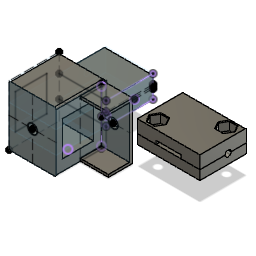
cessna-throttle-v39 (Autodesk Fusion 360 design; units mm, degrees)
Autodesk Fusion 360 part; units mm, degrees
note: some values were not read from the file. Chosen so that the rebuilt part matches the saved one: which bodies a step acts on.
sketch "Sketch1" plane through (0, 0, 0) normal (0, 1, 0) x (1, 0, 0)
  line L0 (0, 0) -> (20, 0)
  line L1 (20, 0) -> (20, 15)
  line L2 (20, 15) -> (0, 15)
  line L3 (0, 15) -> (0, 0)
  line L4 (6, 0) -> (6, 7)
  line L5 (6, 7) -> (14, 7)
  line L6 (14, 7) -> (14, 0)
  line L7 (10, 15) -> (10, 0) construction
  line L8 (0, 10) -> (20, 10) construction
  line L9 (20, 10) -> (20, 8.05) construction
  line L10 (20, 8.05) -> (0, 8.05) construction
  line L11 (0, 8.05) -> (0, 10) construction
  circle A0 centre (3.5, 3.05) radius 1
  circle A1 centre (16.5, 12) radius 1
  dimension "d1" = 7
  dimension "d2" = 8
  dimension "d3" = 20
  dimension "d4" = 15
  dimension "d5" = 1.95
  dimension "d6" = 5
  dimension "d7" = 2
  dimension "d8" = 3.5
  dimension "d9" = 5
  dimension "d10" = 2
  dimension "d11" = 2
  dimension "d12" = 3.5
  constraint horizontal L0
  constraint vertical L1
  constraint horizontal L2
  constraint vertical L3
  constraint coincident L0 L4.start
  constraint perpendicular L0 L4
  constraint perpendicular L4 L5
  constraint coincident L0 L6.end
  constraint perpendicular L0 L6
  constraint midpoint L2 L7.start
  constraint midpoint L0 L7.end
  constraint symmetric L4.end L5.end L7
  constraint coincident L0.start L3.end
  constraint horizontal L8
  constraint vertical L9
  constraint horizontal L10
  constraint vertical L11
  constraint coincident L1 L9.end
  constraint coincident L3 L8.start
  measures "d1" distance of L4.start L4.end
  measures "d2" distance of L4.end L5.end
  measures "d3" distance of L1.end L2.end
  measures "d4" distance of L0.start L2.end
  measures "d5" distance of L8 L10
  measures "d6" distance of L2 L8
  measures "d7" diameter of A0
  measures "d8" distance of L3 A0.centre
  measures "d9" distance of L10 A0.centre
  measures "d10" diameter of A1
  measures "d11" distance of L8 A1.centre
  measures "d12" distance of L1 A1.centre
extrude "Extrude1" add sketch "Sketch1" along normal blind 1.12 contours L0 L1 L2 L3 L4 L5 L6 makes body 1
sketch "Sketch2" plane through (0, 1.12, 0) normal (0, 1, 0) x (-1, 0, 0)
  circle A0 centre (-16.5, -12) radius 1
  circle A1 centre (-3.5, -3.05) radius 1
  line L0 (-14, -7) -> (-14, 0)
  line L1 (-14, 0) -> (-20, 0)
  line L2 (-20, 0) -> (-20, -15)
  line L3 (-20, -15) -> (0, -15)
  line L4 (0, -15) -> (0, 0)
  line L5 (0, 0) -> (-6, 0)
  line L6 (-6, 0) -> (-6, -7)
  line L7 (-6, -7) -> (-14, -7)
  line L8 (0, -15) -> (-20, -15)
  line L9 (-20, -15) -> (-20, 0)
  line L10 (-20, 0) -> (0, 0)
  line L11 (0, 0) -> (0, -15)
  constraint horizontal L8
  constraint vertical L9
  constraint horizontal L10
  constraint vertical L11
  constraint coincident L1.end L2.start
  constraint coincident L3.end L4.start
extrude "Extrude2" add sketch "Sketch2" along normal blind 3 bodies 1
sketch "Sketch3" plane through (0, 0, 0) normal (0, -1, 0) x (1, 0, 0)
  circle A0 centre (16.5, -12) radius 1
  circle A1 centre (3.5, -3.05) radius 1
  line L0 (14, 0) -> (14, -7)
  line L1 (14, -7) -> (6, -7)
  line L2 (6, -7) -> (6, 0)
  line L3 (6, 0) -> (0, 0)
  line L4 (0, 0) -> (0, -15)
  line L5 (0, -15) -> (20, -15)
  line L6 (20, -15) -> (20, 0)
  line L7 (20, 0) -> (14, 0)
  line L8 (0, 0) -> (20, 0)
  line L9 (20, 0) -> (20, -15)
  line L10 (20, -15) -> (0, -15)
  line L11 (0, -15) -> (0, 0)
  constraint horizontal L8
  constraint vertical L9
  constraint horizontal L10
  constraint vertical L11
  constraint coincident L5.end L6.start
  constraint coincident L3.end L4.start
extrude "Extrude3" add sketch "Sketch3" along normal blind 3 bodies 1
sketch "Sketch4" plane through (0, 0, 0) normal (-1, 0, 0) x (0, 0, 1)
  line L0 (0, -3) -> (0, 4.12)
  line L1 (0, 4.12) -> (-15, 4.12)
  line L2 (-15, 4.12) -> (-15, -3)
  line L3 (-15, -3) -> (0, -3)
  circle A0 centre (-9.025, 0) radius 0.975
  line L4 (-15, 0) -> (0, 0)
  point P0 (-10, 0)
  point P1 (-8.05, 0)
  constraint coincident P0 A0
  constraint coincident P1 A0
  constraint coincident A0.centre L4
extrude "Extrude4" cut sketch "Sketch4" against normal blind 25 contours A0 L4 | A0 L4 bodies 1
sketch "Sketch5" plane through (0, -3, 0) normal (0, -1, 0) x (1, 0, 0)
  circle A0 centre (16.5, -12) radius 1
  circle A1 centre (3.5, -3.05) radius 1
  line L0 (0, -15) -> (20, -15)
  line L1 (20, -15) -> (20, 0)
  line L2 (20, 0) -> (0, 0)
  line L3 (0, 0) -> (0, -15)
  circle A2 centre (3.5, -3.05) radius 1.75
  circle A3 centre (16.5, -12) radius 1.75
  dimension "d21" = 3.5
  dimension "d22" = 3.5
  constraint concentric A1 A2
  constraint concentric A0 A3
  measures "d21" diameter of A2
  measures "d22" diameter of A3
extrude "Extrude5" cut sketch "Sketch5" against normal blind 1.7 contours A2 | A3 bodies 1
sketch "Sketch6" plane through (0, 4.12, 0) normal (0, 1, 0) x (-1, 0, 0)
  circle A0 centre (-16.5, -12) radius 1
  circle A1 centre (-3.5, -3.05) radius 1
  line L0 (0, 0) -> (-20, 0)
  line L1 (-20, 0) -> (-20, -15)
  line L2 (-20, -15) -> (0, -15)
  line L3 (0, -15) -> (0, 0)
  line L4 (-15.25, -14.1651) -> (-14, -12)
  line L5 (-14, -12) -> (-15.25, -9.8349)
  line L6 (-15.25, -9.8349) -> (-17.75, -9.8349)
  line L7 (-17.75, -9.8349) -> (-19, -12)
  line L8 (-19, -12) -> (-17.75, -14.1651)
  line L9 (-17.75, -14.1651) -> (-15.25, -14.1651)
  line L10 (-20, -15) -> (0, -15)
  line L11 (-2.25, -5.2151) -> (-1, -3.05)
  line L12 (-1, -3.05) -> (-2.25, -0.8849)
  line L13 (-2.25, -0.8849) -> (-4.75, -0.8849)
  line L14 (-4.75, -0.8849) -> (-6, -3.05)
  line L15 (-6, -3.05) -> (-4.75, -5.2151)
  line L16 (-4.75, -5.2151) -> (-2.25, -5.2151)
  line L17 (0, 0) -> (-20, 0)
  point P0 (-16.5, -12)
  point P1 (-3.5, -3.05)
  dimension "d25" = 2.5
  dimension "d26" = 2.5
  constraint coincident P0 A0.centre
  constraint parallel L9 L10
  constraint coincident P1 A1.centre
  constraint parallel L16 L17
  measures "d25" distance of L4.start P0
  measures "d26" distance of L11.start P1
extrude "Extrude6" cut sketch "Sketch6" against normal blind 2.8 contours L4 L5 L6 L7 L8 L9 | L11 L12 L13 L14 L15 L16 bodies 1
ref_plane "WorkPlane1" through (-10, 0.56, -7.5) normal (-1, 0, 0) x (0, 0, 1)
sketch "Sketch7" plane through (-10, 0.56, -7.5) normal (-1, 0, 0) x (0, 0, -1)
  circle A0 centre (1.525, 0.56) radius 0.975
  line L0 (-7.5, 3.56) -> (-7.5, -3.56)
  line L1 (-7.5, -3.56) -> (7.5, -3.56)
  line L2 (7.5, -3.56) -> (7.5, 3.56)
  line L3 (7.5, 3.56) -> (-7.5, 3.56)
  circle A1 centre (1.525, 0.56) radius 1.05
  dimension "d32" = 2.1
  constraint concentric A0 A1
  measures "d32" diameter of A1
extrude "Extrude7" add sketch "Sketch7" along normal blind 15 separate body contours L0 L1 L2 L3 makes body 2
split "Split1" by plane through (0, 0, 0) normal (0, 1, 0) bodies 1 makes body 3 at (13.75, 4.12, -4.295)
extrude "Extrude8" add 1 faces at (-15, -0.6267, 0) along direction (0, 0, 1) blind 16 on bodies 2 bodies 2
sketch "Sketch8" plane through (0, 4.12, 0) normal (0, 1, 0) x (-1, 0, 0)
  line L0 (10, 16) -> (10, -15)
  line L1 (10, -15) -> (25, -15)
  line L2 (25, -15) -> (25, 16)
  line L3 (25, 16) -> (10, 16)
  line L4 (10, 0) -> (25, 0)
  point P0 (10, 0)
  constraint coincident P0 L4.start
  constraint coincident L2 L4.end
  constraint perpendicular L2 L4
extrude "Extrude9" add sketch "Sketch8" along normal blind 6 contours L0 L2 L3 L4 bodies 2
sketch "Sketch9" plane through (0, -3, 0) normal (0, -1, 0) x (1, 0, 0)
  line L0 (-10, -15) -> (-10, 16)
  line L1 (-10, 16) -> (-25, 16)
  line L2 (-25, 16) -> (-25, -15)
  line L3 (-25, -15) -> (-10, -15)
  line L4 (-10, 0) -> (-25, 0)
  point P0 (-10, 0)
  constraint coincident P0 L4.start
  constraint coincident L2 L4.end
  constraint perpendicular L2 L4
extrude "Extrude10" add sketch "Sketch9" along normal blind 6 contours L0 L1 L2 L4 bodies 2
sketch "Sketch10" plane through (-25, 0, 0) normal (-1, 0, 0) x (0, 0, 1)
  circle A0 centre (-9.025, 0) radius 1.05
  line L0 (-15, -3) -> (0, -3)
  line L1 (0, -3) -> (0, -9)
  line L2 (0, -9) -> (16, -9)
  line L3 (16, -9) -> (16, 10.12)
  line L4 (16, 10.12) -> (0, 10.12)
  line L5 (0, 10.12) -> (0, 4.12)
  line L6 (0, 4.12) -> (-15, 4.12)
  line L7 (-15, 4.12) -> (-15, -3)
  line L8 (0, 10.12) -> (16, 10.12) construction
  line L9 (16, 10.12) -> (16, -9) construction
  line L10 (16, -9) -> (0, -9) construction
  line L11 (0, -9) -> (0, 10.12) construction
  line L12 (4, 6.12) -> (14, 6.12)
  line L13 (14, 6.12) -> (14, -5)
  line L14 (14, -5) -> (4, -5)
  line L15 (4, -5) -> (4, 6.12)
  dimension "d39" = 2
  dimension "d40" = 4
  dimension "d41" = 4
  dimension "d42" = 4
  constraint horizontal L8
  constraint vertical L9
  constraint horizontal L10
  constraint vertical L11
  constraint coincident L2.end L3.start
  constraint coincident L4.end L5.start
  constraint horizontal L12
  constraint vertical L13
  constraint horizontal L14
  constraint vertical L15
  measures "d39" distance of L9 L13
  measures "d40" distance of L11 L15
  measures "d41" distance of L8 L12
  measures "d42" distance of L10 L14
extrude "Extrude11" cut sketch "Sketch10" against normal blind 15 contours L12 L13 L14 L15 bodies 2
fillet "Fillet1" radius 0.2 12 edges at (14.625, 4.12, -13.0825) (16.5, 4.12, -14.1651) (18.375, 4.12, -13.0825) (18.375, 4.12, -10.9175) (16.5, 4.12, -9.8349) (14.625, 4.12, -10.9175) (3.5, 4.12, -5.2151) (5.375, 4.12, -4.1325) (5.375, 4.12, -1.9675) (3.5, 4.12, -0.8849) (1.625, 4.12, -1.9675) (1.625, 4.12, -4.1325) on bodies 3
fillet "Fillet2" radius 0.5 14 edges at (10, -3, -15) (-17.5, 10.12, 0) (-17.5, -9, 0) (-17.5, -3, -15) (-17.5, 4.12, -15) (-10, -6, 0) (-25, -6, 0) (-10, 7.12, 0) (-25, 7.12, 0) (-10, 10.12, 8) (-25, 10.12, 8) (-10, -9, 8) (-25, -9, 8) (10, 4.12, -15) on bodies 1 2 3
sketch "Sketch11" plane through (-10, 0, 0) normal (1, 0, 0) x (0, 0, -1)
  arc A0 (15, 3.62) -> (14.5, 4.12) centre (14.5, 3.62) ccw
  line L0 (14.5, 4.12) -> (-0.5, 4.12)
  line L1 (-0.5, 4.12) -> (-0.5, 9.62)
  line L2 (-0.5, 9.62) -> (-16, 9.62)
  line L3 (-16, 9.62) -> (-16, -8.5)
  line L4 (-16, -8.5) -> (-0.5, -8.5)
  line L5 (-0.5, -8.5) -> (-0.5, -3)
  line L6 (-0.5, -3) -> (14.5, -3)
  arc A1 (14.5, -3) -> (15, -2.5) centre (14.5, -2.5) ccw
  line L7 (15, -2.5) -> (15, 3.62)
  circle A2 centre (9.025, 0) radius 1.05
  line L8 (-14, -5) -> (-14, 6.12)
  line L9 (-14, 6.12) -> (-4, 6.12)
  line L10 (-4, 6.12) -> (-4, -5)
  line L11 (-4, -5) -> (-14, -5)
  line L12 (-1.5, 9.62) -> (-1.5, -8.5) construction
  line L13 (0, 1.12) -> (15, 1.12) construction
  line L14 (0, 0) -> (15, 0) construction
  line L15 (15, 0.56) -> (-1.5, 0.56) construction
  line L16 (-8.28, 8.81) -> (-1.5, 8.81) construction
  line L17 (-1.5, 8.81) -> (-1.5, -7.69) construction
  line L18 (-1.5, -7.69) -> (-8.28, -7.69) construction
  line L19 (-8.28, -7.69) -> (-8.28, 8.81) construction
  line L20 (-8.28, 8.81) -> (-8.28, 9.61)
  line L21 (-8.28, 9.61) -> (0, 9.61)
  line L22 (0, 9.61) -> (0, -8.5)
  line L23 (0, -8.5) -> (-8.25, -8.5)
  line L24 (-8.25, -8.5) -> (-8.28, -7.69)
  line L25 (-8.28, -7.69) -> (-1.5, -7.69)
  line L26 (-1.5, -7.69) -> (-1.5, 8.81)
  line L27 (-1.5, 8.81) -> (-8.28, 8.81)
  point P0 (0, 1.12)
  point P1 (15, 1.12)
  point P2 (15, 0)
  dimension "d47" = 1
  dimension "d48" = 6.78
  dimension "d49" = 16.5
  dimension "d50" = 0.8
  dimension "d51" = 8.28
  constraint coincident L2 L12.start
  constraint coincident L4 L12.end
  constraint perpendicular L4 L12
  constraint coincident P0 L13.start
  constraint coincident P1 L13.end
  constraint coincident L14.start origin
  constraint coincident P2 L14.end
  constraint coincident L7 L15.start
  constraint coincident L12 L15.end
  constraint perpendicular L12 L15
  constraint symmetric P1 P2 L15
  constraint horizontal L16
  constraint vertical L17
  constraint horizontal L18
  constraint vertical L19
  constraint collinear L12 L17
  constraint symmetric L15 L16.end L17.end
  constraint perpendicular L16 L20
  constraint parallel L2 L21
  constraint perpendicular L6 L22
  constraint midpoint L4 L23.end
  constraint perpendicular L5 L23
  measures "d47" distance of L1 L12
  measures "d48" distance of L16.start L16.end
  measures "d49" distance of L16.start L18.end
  measures "d50" distance of L16.start L20.end
  measures "d51" horizontal distance of L20.end L21.end
extrude "Extrude12" add sketch "Sketch11" along normal blind 9 contours L0 L1 L4 L5 L6 L20 L21 L22 L23 L24 L25 L26 L27 | L0 L1 L21 L22 | L5 L6 L22 L23 bodies 2
sketch "Sketch12" plane through (0, 0, 1.5) normal (0, 0, 1) x (1, 0, 0)
  line L0 (-10, 8.81) -> (-10, -7.69)
  line L1 (-10, -7.69) -> (-1, -7.69)
  line L2 (-1, -7.69) -> (-1, 8.81)
  line L3 (-1, 8.81) -> (-10, 8.81)
  line L4 (-10, 0.56) -> (-1, 0.56) construction
  circle A0 centre (-6.2, 0.56) radius 1.5
  line L5 (-10, 8.81) -> (-10, -7.69) construction
  point P0 (-10, 0.56)
  dimension "d55" = 3
  dimension "d56" = 3.8
  constraint coincident P0 L4.start
  constraint midpoint L2 L4.end
  constraint coincident L4 A0.centre
  measures "d55" diameter of A0
  measures "d56" distance of A0.centre L5
extrude "Extrude15" cut 1 faces at (-4, -0.63, 0) along direction (0, 0, 1) blind 0.5 on bodies 2 bodies 2
extrude "Extrude13" cut sketch "Sketch12" against normal blind 2 contours A0 bodies 2
sketch "Sketch13" plane through (0, 0, 16) normal (0, 0, 1) x (1, 0, 0)
  arc A0 (-10.5, -9) -> (-10, -8.5) centre (-10.5, -8.5) ccw
  line L0 (-10, -8.5) -> (-10, 9.62)
  arc A1 (-10, 9.62) -> (-10.5, 10.12) centre (-10.5, 9.62) ccw
  line L1 (-10.5, 10.12) -> (-24.5, 10.12)
  arc A2 (-24.5, 10.12) -> (-25, 9.62) centre (-24.5, 9.62) ccw
  line L2 (-25, 9.62) -> (-25, -8.5)
  arc A3 (-25, -8.5) -> (-24.5, -9) centre (-24.5, -8.5) ccw
  line L3 (-24.5, -9) -> (-10.5, -9)
  circle A4 centre (-17.5, 0.56) radius 1.5
  line L4 (-17.5, 10.12) -> (-17.5, -9) construction
  line L5 (-25, 0.56) -> (-10, 0.56) construction
  point P0 (-6.2, 0.56)
  dimension "d59" = 3
  constraint midpoint L1 L4.start
  constraint midpoint L3 L4.end
  constraint midpoint L2 L5.start
  constraint midpoint L0 L5.end
  constraint coincident A4.centre L4
  constraint coincident A4.centre L5
  measures "d59" diameter of A4
extrude "Extrude14" cut sketch "Sketch13" against normal blind 2 contours A4 bodies 2
equation "d51 = 6.78 mm + 1.5 mm"
